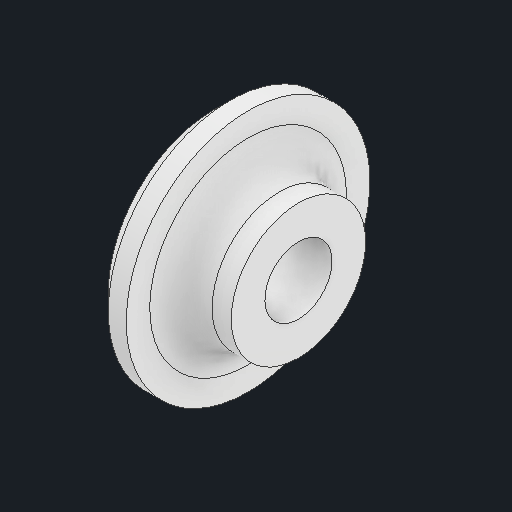
# Autodesk Inventor part: 축종아리베어링고정
Saved by Autodesk Inventor 2027.1 (Build 311270010, 270A)
## iProperties
Created: 2026-08-20
Part Number: 축종아리베어링고정
Material: ABS 플라스틱
Document SubType Name: Modeling
Designer: moieboy9999
Density: 1.06 g/cm^3
Appearance: 매끄러움 - 흰색
Mass: 0.303228 g
Surface Area: 3.7703 cm^2
Volume: 0.286065 cm^3
Author: moieboy9999
## iProperties of the stored document 축종아리베어링고정_3D 인쇄.ipt
Created: 2026-08-21
Part Number: 축종아리베어링고정_3D 인쇄
Material: 일반
Document SubType Name: Modeling
Designer: maker
Density: 1 g/cm^3
Appearance: 기본값
Author: maker
Autodesk Inventor part; units mm, degrees
ref_plane "YZ Plane" through (0, 0, 0) normal (1, 0, 0) x (0, 1, 0)
ref_plane "XZ Plane" through (0, 0, 0) normal (0, 1, 0) x (-1, 0, 0)
ref_plane "XY Plane" through (0, 0, 0) normal (0, 0, 1) x (1, 0, 0)
sketch "스케치1" plane through (0, 0, 0) normal (1, 0, 0) x (0, 1, 0)
  circle A0 centre (0, 0) radius 6.5
  circle A1 centre (0, 0) radius 1.75
  circle A2 centre (0, 0) radius 3.5
  dimension "d0" = 13
  dimension "d1" = 3.5
  dimension "d2" = 7
  constraints: 3 centre point, 3 coincident
  measures "d0" diameter of A0
  measures "d1" diameter of A1
  measures "d2" diameter of A2
extrude "돌출1" add sketch "스케치1" against normal blind 2 contours A0 | A2
extrude "돌출2" add sketch "스케치1" along normal blind 2.625 contours A2
fillet "모깎기1" radius 1.625 1 edges at (0, -3.5, 0)
chamfer "모따기1" distance 1 angle 45 1 edges at (-2, -6.5, 0)
move faces "이동1" translate (0.2, 0, 0) faces at (-2, 4.1798, -0.5783)
offset faces "크기2" outward -0.15 faces at (-0.3333, 6.4789, -0.523) (-1.2667, -2.6722, -5.6315)
